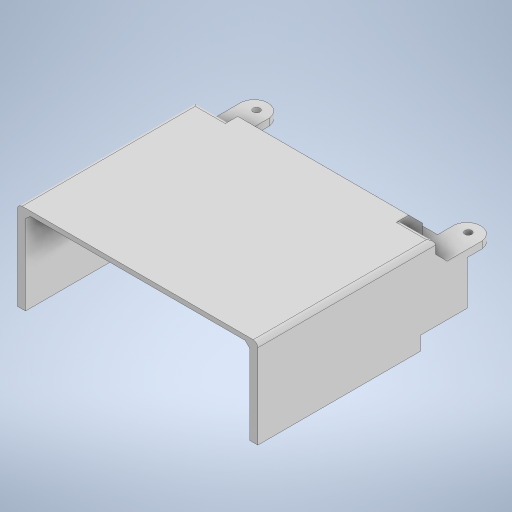
# Autodesk Inventor part: tampa_principal_v2
Saved by Autodesk Inventor 2024.3 (Build 283343000, 343)
## iProperties
Created: 2025-02-24
Part Number: tampa_principal_v2
Material: Genérico
Document SubType Name: Modeling
Designer: lostv
Density: 1 g/cm^3
Appearance: Padrão
Author: lostv
Autodesk Inventor part; units mm, degrees
ref_plane "YZ Plane" through (0, 0, 0) normal (1, 0, 0) x (0, 1, 0)
ref_plane "XZ Plane" through (0, 0, 0) normal (0, 1, 0) x (-1, 0, 0)
ref_plane "XY Plane" through (0, 0, 0) normal (0, 0, 1) x (1, 0, 0)
sketch "Esboço1" plane through (0, 0, 0) normal (0, 1, 0) x (-1, 0, 0)
  line L0 (-64.0697, 52.888) -> (39.938, 52.888)
  line L1 (39.938, 52.888) -> (39.938, -22.879)
  line L2 (24.9381, -35.9271) -> (-49.0698, -35.9078)
  line L3 (24.9381, -35.9271) -> (24.9376, -22.982)
  line L4 (-49.0698, -35.9078) -> (-49.0703, -22.982)
  line L5 (27.9858, -33.9511) -> (28.0265, -22.9819)
  line L6 (-60.5085, -22.8381) -> (-60.5908, -38.1314) construction
  line L7 (39.938, -22.879) -> (39.938, -40.2377)
  circle A0 centre (-57.062, -28.879) radius 1.75
  circle A1 centre (32.938, -28.879) radius 1.75
  circle A2 centre (33.72, -46.8489) radius 1.5
  circle A3 centre (20.938, -31.0333) radius 1.75
  line L8 (24.9409, -35.9271) -> (24.9409, -22.982)
  circle A4 centre (-45.062, -31.0333) radius 1.75
  line L9 (-49.0698, -35.9271) -> (-49.0703, -22.982)
  circle A5 centre (-57.9167, -46.8032) radius 1.5
  ellipse E0 centre (-12.062, -134.482) end of major axis (91.4418, -134.482) minor radius 109.0041 (-49.07, -32.6838) -> (-64.0697, -40.2377) ccw
  ellipse E1 centre (-12.062, -134.482) end of major axis (91.438, -134.482) minor radius 109 (39.938, -40.2377) -> (24.938, -32.6849) ccw
  line L10 (-26.1851, -35.9201) -> (-26.1736, -35.9138)
  line L11 (2.0613, -35.9201) -> (2.0632, -35.9211)
  line L12 (36.438, -41.6421) -> (36.4459, -41.6535)
  line L13 (-60.6095, -41.6063) -> (-60.624, -41.6211)
  line L14 (29.938, -22.9847) -> (29.938, -22.982)
  line L15 (36.4326, -22.982) -> (36.4326, 52.888)
  line L16 (-60.5537, -22.982) -> (-60.5537, 52.888)
  line L17 (39.938, 50.388) -> (-64.0697, 50.388)
  line L18 (39.938, -19.982) -> (36.4326, -19.982)
  line L19 (39.938, -22.982) -> (-64.0697, -22.982)
  line L20 (-60.5537, -19.982) -> (-64.0697, -19.982)
  line L21 (-64.0697, -40.2377) -> (-64.0697, -46.7789)
  line L22 (-64.0697, -46.7789) -> (-52.1176, -46.7789)
  arc A6 (-64.0697, -46.7789) -> (-52.1176, -46.7789) centre (-58.0936, -45.9872) ccw
  line L23 (-12.0659, -35.9174) -> (-12.0659, 0) construction
  line L24 (39.938, -40.2377) -> (39.938, -46.7789)
  line L25 (39.938, -46.7789) -> (27.9858, -46.7789)
  arc A7 (27.9858, -46.7789) -> (39.938, -46.7789) centre (33.9619, -45.9872) ccw
  line L26 (-52.1176, -46.7789) -> (-52.1176, -22.982)
  line L27 (27.9858, -46.7789) -> (27.9858, -33.9511)
  line L28 (-52.1176, -39.337) -> (27.9858, -39.337)
  line L29 (-64.0697, -40.2377) -> (-64.0697, 52.888)
  line L30 (39.938, -26.5255) -> (24.9409, -26.5261)
  line L31 (-49.0702, -26.5289) -> (-64.0697, -26.5295)
  point P0 (0, 0)
  point P1 (-13.31, 23.8291)
  point P2 (-12.062, -22.982)
  point P3 (63.9356, 48.927)
  point P4 (59.9356, 42.927)
  point P5 (-12.062, -28.482)
  point P6 (-12.062, -22.982)
  point P7 (-52.07, -35.7208)
  point P8 (-52.07, -28.4726)
  point P9 (-49.0701, -29.4449)
  point P10 (-52.0701, -30.1013)
  point P11 (24.9409, -32.6849)
  point P12 (-49.07, -32.666)
  point P13 (24.9409, -29.4545)
  point P14 (-49.0701, -29.4545)
  point P15 (-54.1562, -51.2802)
  point P16 (36.4326, 50.388)
  point P17 (-60.5537, 50.388)
  point P18 (38.1853, -19.982)
  point P19 (-12.062, -22.982)
  point P20 (-60.5566, -22.982)
  point P21 (36.4326, -22.982)
  point P22 (28.0265, -22.982)
  point P23 (27.938, -33.9512)
  point P24 (24.9376, -22.982)
  point P25 (-49.0703, -22.982)
  point P26 (-49.07, -22.982)
  point P27 (24.9376, -22.982)
  point P28 (-49.0703, -22.982)
  point P29 (27.9858, -33.9723)
  point P30 (-49.0703, -22.982)
  point P31 (-64.0697, -19.982)
  point P32 (-60.5537, -22.982)
  point P33 (-52.1176, -33.9713)
  point P34 (-64.0697, 50.388)
  point P35 (24.9409, -22.982)
  point P36 (24.9409, -32.6861)
  dimension "d2" = 3
  dimension "d6" = 66
  dimension "d16" = 3.5054
  dimension "d18" = 2.5
  dimension "d27" = 12.9451
  dimension "d28" = 88.8152
  dimension "d29" = 3
  constraints: 64 end point, 23 point on line, 9 perpendicular, 8 centre point, 6 vertical, 5 midpoint, 4 horizontal, 4 point on circle, 4 symmetric about line, 1 collinear, 9 other
  measures "d2" horizontal distance of point (-49.07, -29.445) point (-52.07, -30.101)
  measures "d6" distance of A3.centre A4.centre
  measures "d16" distance between parallel lines of L15 L1
  measures "d18" distance between parallel lines of L0 L17
  measures "d27" distance of L8.end L2.start
  measures "d28" distance from line of L0 L8.start
  measures "d29" distance between parallel lines of L19 L18
extrude "Extrusão1" add sketch "Esboço1" against normal blind 2 contours L17 L15 L19 L16
extrude "Extrusão2" add sketch "Esboço1" against normal blind 38.5 contours L17 L16 L20 L29 | L17 L1 L18 L15
extrude "Extrusão3" add sketch "Esboço1" against normal blind 32.5 contours L20 L16 L19 L29 | L19 L26 L31 L29 | L18 L1 L7 L19 L15 | L31 L26 E0 L29 | L19 L7 L30 L5 | L7 E1 L27 L5 L30
extrude "Extrusão4" add sketch "Esboço1" against normal blind 13.5 contours L19 L26 L31 L29 | L31 L26 E0 L29 | L19 L7 L30 L5 | L19 L4 L31 L26 | E0 L26 L22 A5 L21 | L31 L4 E0 L26 | L19 L3 L2 L4 | E0 L4 L2 L3 E1 L27 L28 L26 | L22 A5 A6 | L7 E1 L27 L5 L30 | L5 L30 L8 L19 | L19 L8 E1 L3 | L24 L25 A2 L27 E1 | L5 L27 E1 L8 L30 | A7 L25 A2 | A0 | A1 | A3 | A4
extrude "Extrusão5" cut sketch "Esboço1" against normal blind 10.5 contours L31 L26 E0 L29 | E0 L26 L22 A5 L21 | L31 L4 E0 L26 | E0 L4 L2 L3 E1 L27 L28 L26 | L22 A5 A6 | L7 E1 L27 L5 L30 | L22 A5 | A5 L22 | L24 L25 A2 L27 E1 | L5 L27 E1 L8 L30 | A7 L25 A2 | L25 A2 | A2 L25 | A0 | A1
chamfer "Chanfro1" distance 6 angle 45 3 edges at (-26.4821, -13.5, -22.982) (50.5939, -13.5, -22.982) (12.0659, 0, -35.9174)
chamfer "Chanfro3" distance 5 angle 45 1 edges at (12.0455, -7.5, -22.982)
chamfer "Chanfro4" distance 3 angle 45 1 edges at (12.0567, -13.5, -28.982)
chamfer "Chanfro6" distance 2 angle 45 2 edges at (-36.4326, -2, 13.703) (60.5537, -2, 13.703)
fillet "Arredondamento1" radius 2 4 edges at (64.0697, 0, 11.9293) (56.57, 0, -26.5292) (-32.4394, 0, -26.5258) (-39.938, 0, 11.9313)
chamfer "Chanfro7" distance 5 angle 45 2 edges at (56.57, -10.5, -26.5292) (-32.4394, -10.5, -26.5258)
